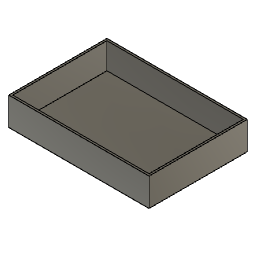
Conatiner 2 v2 (Autodesk Fusion 360 design; units mm, degrees)
Autodesk Fusion 360 part; units mm, degrees
sketch "Sketch1" plane through (0, 0, 0) normal (0, 0, 1) x (1, 0, 0)
  line L0 (63.375, 42.565) -> (-63.375, 42.565)
  line L1 (-63.375, 42.565) -> (-63.375, -42.565)
  line L2 (-63.375, -42.565) -> (63.375, -42.565)
  line L3 (63.375, -42.565) -> (63.375, 42.565)
  line L4 (63.375, 42.565) -> (-63.375, -42.565) construction
  line L5 (-63.375, 42.565) -> (63.375, -42.565) construction
  line L6 (-68.375, 47.565) -> (68.375, 47.565)
  line L7 (68.375, 47.565) -> (68.375, -47.565)
  line L8 (68.375, -47.565) -> (-68.375, -47.565)
  line L9 (-68.375, -47.565) -> (-68.375, 47.565)
  line L10 (-68.375, 47.565) -> (68.375, -47.565) construction
  line L11 (68.375, 47.565) -> (-68.375, -47.565) construction
  line L12 (71.5, 47.565) -> (68.5, 47.565)
  line L13 (68.5, 47.565) -> (68.5, -47.565)
  line L14 (68.5, -47.565) -> (71.5, -47.565)
  line L15 (71.5, -47.565) -> (71.5, 47.565)
  line L16 (71.5, 47.565) -> (68.5, -47.565) construction
  line L17 (68.5, 47.565) -> (71.5, -47.565) construction
  line L18 (71.4437, -50.4298) -> (-68.3063, -50.4298)
  line L19 (-68.3063, -50.4298) -> (-68.3063, -47.4298)
  line L20 (-68.3063, -47.4298) -> (71.4437, -47.4298)
  line L21 (71.4437, -47.4298) -> (71.4437, -50.4298)
  line L22 (71.4437, -50.4298) -> (-68.3063, -47.4298) construction
  line L23 (-68.3063, -50.4298) -> (71.4437, -47.4298) construction
  point P0 (70, 0)
  point P1 (1.5687, -48.9298)
  dimension "d1" = 126.75
  dimension "d2" = 85.13
  dimension "d3" = 136.75
  dimension "d4" = 95.13
  dimension "d5" = 3
  dimension "d6" = 139.75
  dimension "d7" = 3
  constraint horizontal L0
  constraint perpendicular L0 L1
  constraint parallel L0 L2
  constraint parallel L1 L3
  constraint coincident L4 origin
  constraint coincident L5 origin
  constraint horizontal L6
  constraint perpendicular L6 L7
  constraint parallel L6 L8
  constraint parallel L7 L9
  constraint coincident L10 origin
  constraint coincident L11 origin
  constraint horizontal L12
  constraint perpendicular L12 L13
  constraint parallel L12 L14
  constraint parallel L13 L15
  constraint coincident L16 P0
  constraint coincident L17 P0
  constraint horizontal L18
  constraint perpendicular L18 L19
  constraint parallel L18 L20
  constraint parallel L19 L21
  constraint coincident L22 P1
  constraint coincident L23 P1
  measures "d1" distance of L1.end L2.end
  measures "d2" distance of L0.end L1.end
  measures "d3" distance of L7.end L8.end
  measures "d4" distance of L6.end L7.end
  measures "d5" distance of L13.end L14.end
  measures "d6" distance of L19.end L20.end
  measures "d7" distance of L18.end L19.end
sketch "Sketch2" plane through (0, 0, 0) normal (0, 0, 1) x (1, 0, 0)
sketch "Sketch3" plane through (0, 0, 0) normal (0, 0, 1) x (1, 0, 0)
  line L0 (71.4782, -50.4736) -> (-68.4999, -50.4736)
  line L1 (-68.4999, -50.4736) -> (-68.4999, 47.4954)
  line L2 (-68.4999, 47.4954) -> (71.4782, 47.4954)
  line L3 (71.4782, 47.4954) -> (71.4782, -50.4736)
  constraint horizontal L0
  constraint vertical L1
  constraint horizontal L2
  constraint vertical L3
extrude "Extrude1" add sketch "Sketch3" along normal blind 28
shell "Shell1" thickness 2 removed faces 1 at (-21.8406, -17.8173, 28)
extrude "Extrude2" add sketch "Sketch1" against normal blind 3 contours L0 L1 L2 L3
extrude "Extrude3" add 1 faces at (-21.125, -14.1883, -3) along direction (0, 0, -1) blind 4.9
